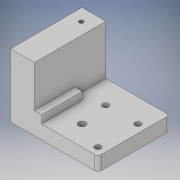
# Autodesk Inventor part: BaseMount
Saved by Autodesk Inventor 2019 (Build 230136000, 136)
## iProperties
Created: 2019-06-10
Part Number: BaseMount
Material: Generic
Document SubType Name: Modeling
Designer: aorfi
Density: 1 g/cm^3
Appearance: Default
Author: aorfi
Autodesk Inventor part; units mm, degrees
ref_plane "YZ Plane" through (0, 0, 0) normal (1, 0, 0) x (0, 1, 0)
ref_plane "XZ Plane" through (0, 0, 0) normal (0, 1, 0) x (-1, 0, 0)
ref_plane "XY Plane" through (0, 0, 0) normal (0, 0, 1) x (1, 0, 0)
sketch "Sketch1" plane through (0, 0, 0) normal (0, 1, 0) x (-1, 0, 0)
  line L0 (-27.5, 22.5) -> (27.5, 22.5)
  line L1 (27.5, 22.5) -> (27.5, -22.5)
  line L2 (27.5, -22.5) -> (-27.5, -22.5)
  line L3 (-27.5, -22.5) -> (-27.5, 22.5)
  line L4 (-27.5, 22.5) -> (27.5, -22.5) construction
  line L5 (27.5, 22.5) -> (-27.5, -22.5) construction
  point P0 (0, 0)
  dimension "d0" = 45
  dimension "d1" = 55
  constraints: 12 end point, 2 midpoint, 2 parallel, 1 horizontal, 1 perpendicular
  measures "d0" distance of L0.end L1.end
  measures "d1" distance of L1.end L2.end
extrude "Extrusion1" add sketch "Sketch1" along normal mid plane 8.763
sketch "Sketch2" plane through (0, 4.3815, 0) normal (0, 1, 0) x (1, 0, 0)
  line L0 (-27.5, -22.5) -> (27.5, -22.5) projected
  line L1 (27.5, -22.5) -> (27.5, 22.5) projected
  point P0 (4.8, -9.8)
  dimension "d11" = 12.7
  dimension "d12" = 22.7
  measures "d11" distance from line of L0 point (4.8, -9.8)
  measures "d12" distance from line of L1 point (4.8, -9.8)
hole "Hole1" at (4.8, 4.3815, 9.8) direction (0, -1, 0) diameter 4.496 end through all clearance for "Flat Head Machine Screw (82)" size "#8" standard "Ansi Unified Screw Threads"
sketch "Sketch3" plane through (0, 4.3815, 0) normal (0, 1, 0) x (1, 0, 0)
  line L0 (27.5, 22.5) -> (-27.5, 22.5) projected
  line L1 (-27.5, 22.5) -> (-12.5, 22.5)
  line L2 (-12.5, 22.5) -> (-12.5, -22.5)
  line L3 (-12.5, -22.5) -> (-27.5, -22.5)
  line L4 (-27.5, -22.5) -> (-27.5, 22.5)
  line L5 (-27.5, -22.5) -> (27.5, -22.5) projected
  point P0 (0, 0)
  dimension "d13" = 15
  constraints: 8 end point, 2 parallel, 1 collinear, 1 horizontal, 1 perpendicular
  measures "d13" distance of L2.end L3.end
extrude "Extrusion2" add sketch "Sketch3" along normal blind 31.136
sketch "Sketch9" plane through (0, -4.3815, 0) normal (0, -1, 0) x (1, 0, 0)
  circle A0 centre (4.8, 9.8) radius 2.248 projected
  circle A1 centre (4.8, 9.8) radius 4
  point P0 (0, 0)
  dimension "d40" = 8
  constraints: 1 centre point, 1 coincident
  measures "d40" diameter of A1
extrude "Extrusion8" cut sketch "Sketch9" against normal blind 4.318
sketch "Sketch10" plane through (0, -4.3815, 0) normal (0, -1, 0) x (1, 0, 0)
  line L0 (27.5, -22.5) -> (27.5, 22.5) projected
  line L1 (-27.5, -22.5) -> (27.5, -22.5) projected
  line L2 (27.5, 22.5) -> (-27.5, 22.5) projected
  point P0 (0, 0)
  point P1 (22.42, -7.726)
  point P2 (22.42, 17.42)
  point P3 (2.1, -7.726)
  dimension "d43" = 5.08
  dimension "d45" = 20.32
  dimension "d46" = 25.146
  dimension "d65" = 5.08
  constraints: 1 horizontal alignment, 1 vertical alignment
  measures "d43" distance from line of L0 point (22.42, -7.726)
  measures "d45" distance of point (2.1, -7.726) point (22.42, -7.726)
  measures "d46" distance of point (22.42, -7.726) point (22.42, 17.42)
  measures "d65" distance from line of L2 point (22.42, 17.42)
hole "Hole2" at (22.42, -4.3815, -7.726) at (22.42, -4.3815, 17.42) at (2.1, -4.3815, -7.726) direction (0, 1, 0) diameter 3.797 end through all clearance for "Flat Head Machine Screw (82)" size "#6" standard "Ansi Unified Screw Threads"
fillet "Fillet1" radius 2 2 edges at (27.5, 0, 22.5) (27.5, 0, -22.5)
sketch "Sketch13" plane through (0, 35.5175, 0) normal (0, 1, 0) x (1, 0, 0)
  line L0 (-12.5, 22.5) -> (-27.5, 22.5) projected
  point P0 (0, 0)
  point P1 (-20, 14.5)
  point P2 (-20, 22.5)
  dimension "d74" = 8
  constraints: 1 midpoint, 1 vertical alignment
  measures "d74" distance from line of point (-20, 14.5) L0
hole "Hole4" at (-20, 35.5175, -14.5) direction (0, -1, 0) diameter 2.642 depth 10 tip angle 118 thread size "6-32 UNC" class "2B" standard "ANSI Unified Screw Threads"
sketch "Sketch14" plane through (0, 4.3815, 0) normal (0, 1, 0) x (1, 0, 0)
  line L0 (-12.5, -22.5) -> (-12.5, 22.5) projected
  line L1 (-12.5, -22.5) -> (-7.9, -22.5)
  line L2 (-7.9, -22.5) -> (-7.9, 2.9)
  line L3 (-7.9, 2.9) -> (-12.5, 2.9)
  line L4 (-12.5, 2.9) -> (-12.5, -22.5)
  point P0 (0, 0)
  dimension "d89" = 25.4
  dimension "d90" = 4.6
  constraints: 8 end point, 2 parallel, 1 horizontal, 1 perpendicular
  measures "d89" distance of L1.end L2.end
  measures "d90" distance of L2.end L3.end
extrude "Extrusion11" add sketch "Sketch14" along normal blind 5
equation "\"d65\" = d43"
body "Solid1"
